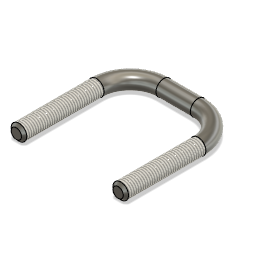
0.883.8395 - Etrier de fixation - IGTE21400_17 Rép. 76 (Autodesk Fusion 360 design; units mm, degrees)
Autodesk Fusion 360 part; units mm, degrees
note: some values were not read from the file. Chosen so that the rebuilt part matches the saved one: how an offset face is resized.
sketch "Sketch1" plane through (0, 0, 0) normal (0, 0, 1) x (1, 0, 0)
  line L0 (0, 0) -> (38.5, 0) construction
  line L1 (0, 0) -> (-38.5, 0) construction
  circle A0 centre (-38.5, 0) radius 6
  circle A1 centre (38.5, 0) radius 6
  dimension "d1" = 38.5
  dimension "d2" = 38.5
  dimension "d9" = 12
  dimension "d10" = 12
  constraint coincident L0.start L1.start
  constraint coincident L1.end A0.centre
  constraint coincident L0.end A1.centre
  measures "d1" distance of L0.start L0.end
  measures "d2" distance of L0.start L1.end
  measures "d9" diameter of A0
  measures "d10" diameter of A1
extrude "Extrude1" add sketch "Sketch1" along normal blind 60 makes body 1 at (-32.5298, -0.5974, 40) makes body 2 at (44.4702, -0.5974, 40)
sketch "Sketch2" plane through (0, 0, 0) normal (0, 1, 0) x (1, 0, 0)
  line L0 (-44.5, -60) -> (-32.5, -60)
  line L1 (-44.5, 0) -> (-32.5, 0)
  line L2 (32.5, -60) -> (44.5, -60)
  line L3 (32.5, 0) -> (44.5, 0)
  line L4 (38.5, 0) -> (38.5, 40) construction
  line L5 (-38.5, 0) -> (-38.5, 0.5) construction
  line L6 (0, 0) -> (0, 20) construction
  line L7 (0, 20) -> (0, 26) construction
  arc A0 (38.5, 0) -> (-38.5, 0) centre (0, -15.5048) ccw construction
  line L8 (0, 26) -> (-13, 26)
  arc A1 (-13, 26) -> (-38.5, 0.5) centre (-13, 0.5) ccw
  arc A2 (38.5, 0.5) -> (13, 26) centre (13, 0.5) ccw
  line L9 (0, 26) -> (13, 26)
  line L10 (-38.5, 0.5) -> (-38.5, 0)
  line L11 (38.5, 0.5) -> (38.5, 0)
  dimension "d13" = 40
  dimension "d15" = 20
  dimension "d16" = 6
  dimension "d24" = 25.5
  constraint midpoint L3 L4.start
  constraint midpoint L1 L5.start
  constraint coincident L6.start origin
  constraint coincident L7.end A0
  constraint tangent A0 L8
  constraint perpendicular L7 L8
  constraint tangent L5 A1
  constraint tangent L8 A1
  constraint symmetric L6 L7.end L8.start
  constraint symmetric L6 L5.end A2.start
  constraint symmetric L6 L8.end A2.end
  constraint symmetric L6 A1 A2
  constraint tangent A2 L11
  measures "d13" distance of L4.start L4.end
  measures "d15" distance of L6.start L6.end
  measures "d16" distance of L6.end L7.end
  measures "d24" radius of A1
sketch "Sketch3" plane through (0, 0, 0) normal (0, 0, -1) x (-1, 0, 0)
  circle A0 centre (38.5, 0) radius 6
  circle A1 centre (38.5, 0) radius 6
  circle A2 centre (38.5, 0) radius 6
sweep "Sweep1" add profiles "Sketch3" path "Sketch2" along L11 A2 L9 L8 A1 L10 section 1 bodies 1 2
thread "Thread1" "ISO Metric profile 12.0 M12x1.75 6g" major diameter 11.8335 minor diameter 9.8365 pitch 1.75 angle 60 resizes the face on face at (-32.5075, -0.2991, 20) on bodies 1
thread "Thread2" "ISO Metric profile 12.0 M12x1.75 6g"
chamfer "Chamfer1" distance 2 angle 45 2 edges at (-44.0163, -2.1396, 60) (32.9837, -2.1396, 60) on bodies 1
equation "d1 = ( 77 / 2 ) * 1 mm"
equation "d2 = ( 77 / 2 ) * 1 mm"
